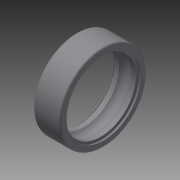
# Autodesk Inventor part: 6201-2Z_PART2
Saved by Autodesk Inventor 2014 SP2 (Build 180246200, 246)
## iProperties
Created: 2019-03-20
Part Number: 6201-2Z_PART2
Material: Generic
Catalog Web Link: www.cadenas.de
Description: -Deep groove ball bearings
Vendor: SKF
Document SubType Name: Modeling
Designer: psadmin
Manufacturer: SKF
Mass: 2.31102 g
Surface Area: 24.4644 cm^2
Volume: 2.31102 cm^3
Density: 1 g/cm^3
Appearance: PSOLRGB-175-175-175
Category: PARTsolutions
Company: SKF
Title: 6201-2Z_PART2
Author: Cadenas PARTsolutions
Comments: Deep groove ball bearings
PSOL_IDENT_0: {$CADENAS_DATA\23d-libs\skf\bearings_units_and_housings\ball_bearings\deep_groove_ball_bearings\bb1_
PSOL_IDENT_1: 001_101.prj},192 {VTYP=3D},{NB=6201-2Z_PART2},{LINA=6201-2Z_PART2},{NN=BB1_001_101_PART2},{NOPRJ=TRU
PSOL_IDENT_2: E},{DATE=18.03.2019 09:24:30},{GEOMDATE=08.08.2018 12:16:40},{VERSION=},{LINEID=9770},{WBVAR=},{WBNU
PSOL_IDENT_3: MERIC=}  {NB=6201-2Z_PART2},{LINA=6201-2Z_PART2},{KT=DUMMY},{PRODUCTID=1050070201},{DESIGNATION=6201
PSOL_IDENT_4: -2Z},{DD=12.00},{D=32.000},{B=10.000},{C=0.000},{DD1=18.45},{DD2=0.0},{D1=0.00},{D2=27.34},{D3=0.00}
PSOL_IDENT_5: ,{D4=0.000},{HH=MIN},{BB=0.000},{FF=0.00},{R0MAX=MIN},{R0=MIN},{R12=0.60},{PITCH=22.00},{DW=6.000},{
PSOL_IDENT_6: DDAMIN=16.200},{DDAMAX=18.400},{DDBMIN=MIN},{DDBMAX=MIN},{DBMIN=MIN},{DAMAX=27.800},{BBAMIN=MIN},{CA
PSOL_IDENT_7: MAX=MIN},{RAMAX=0.600},{LOAD1=7.280},{LOAD2=3.100},{LOAD3=0.132},{SPEED1=50000},{SPEED2=26000},{KR=0
PSOL_IDENT_8: .025},{F0=12.000},{Z=7},{II=1},{MASS=0.039},{BEARING=6201-2Z},{RING=},{HELP=2.990},{HELP2=2.330},{DD
PSOL_IDENT_9: 1ALG=9.225},{YALG=9.225},{PITCH1=22.000},{DW1=6.000},{YALG1=13.010},{HALG1=2.990},{SH=9.225},{CU=0.8
PSOL_IDENT_10: 00},{DESIGN=dgbbw2z},{HALG=3.225},{B1=0},{ALGO=1.000}
NT: Deep groove ball bearings
NB: 6201-2Z_PART2
NBSYN: $DESIGNATION._PART2
LINA: 6201-2Z_PART2
SUPPLIER: SKF
ARTICLENO: 6201-2Z_PART2
BOMINFO: 6201-2Z_PART2
CREATOR: CADENAS GmbH
Autodesk Inventor part; units mm, degrees
ref_plane "YZ Plane" through (0, 0, 0) normal (1, 0, 0) x (0, 1, 0)
ref_plane "XZ Plane" through (0, 0, 0) normal (0, 1, 0) x (-1, 0, 0)
ref_plane "XY Plane" through (0, 0, 0) normal (0, 0, 1) x (1, 0, 0)
sketch "Sketch_17" plane through (0, 0, 0) normal (0, 0, 1) x (1, 0, 0)
  line L0 (50, 0) -> (-50, 0)
  line L1 (0, 15.4) -> (0, 13.67)
  line L2 (0, 13.67) -> (0.18, 13.67)
  arc A0 (0.9, 13.67) -> (0.18, 13.67) centre (0.54, 13.67) ccw
  line L3 (0.9, 13.67) -> (1.0164, 13.01)
  line L4 (1.0164, 13.01) -> (2.7729, 13.01)
  arc A1 (7.2271, 13.01) -> (2.7729, 13.01) centre (5, 11) ccw
  line L5 (7.2271, 13.01) -> (8.9836, 13.01)
  line L6 (8.9836, 13.01) -> (9.1, 13.67)
  arc A2 (9.82, 13.67) -> (9.1, 13.67) centre (9.46, 13.67) ccw
  line L7 (9.82, 13.67) -> (10, 13.67)
  line L8 (10, 13.67) -> (10, 15.4)
  arc A3 (10, 15.4) -> (9.4, 16) centre (9.4, 15.4) ccw
  line L9 (9.4, 16) -> (0.6, 16)
  arc A4 (0.6, 16) -> (0, 15.4) centre (0.6, 15.4) ccw
  constraints: 20 end point, 10 point on circle, 5 centre point
revolve "Revolution1" add sketch "Sketch_17" angle 360 about axis through (50, 0, 0) along (1, 0, 0)
body "Solid1"
